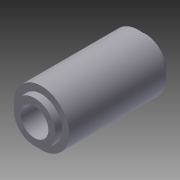
# Autodesk Inventor part: gearbox_standoff
Saved by Autodesk Inventor 2012 (Build 160160000, 160)
## iProperties
Created: 2011-01-16
Part Number: gearbox_standoff
Material: Aluminum-6061
Document SubType Name: Modeling
Designer: Antonella Wilby
Mass: 16.8944 g
Surface Area: 22.1685 cm^2
Volume: 6.23409 cm^3
Density: 2.71 g/cm^3
Author: Antonella Wilby
Autodesk Inventor part; units mm, degrees
ref_plane "YZ Plane" through (0, 0, 0) normal (1, 0, 0) x (0, 1, 0)
ref_plane "XZ Plane" through (0, 0, 0) normal (0, 1, 0) x (-1, 0, 0)
ref_plane "XY Plane" through (0, 0, 0) normal (0, 0, 1) x (1, 0, 0)
sketch "Sketch1" plane through (0, 0, 0) normal (0, 0, 1) x (1, 0, 0)
  circle A0 centre (0, 0) radius 6.35
  circle A1 centre (0, 0) radius 3.175
  dimension "d0" = 12.7
  dimension "d13" = 3.175
  constraints: 2 centre point, 2 coincident
  measures "d0" diameter of A0
  measures "d13" radial gap between concentric circles of A0 A1
extrude "Base" add sketch "Sketch1" along normal mid plane 25.4
sketch "Sketch4" plane through (0, 0, 12.7) normal (0, 0, 1) x (1, 0, 0)
  circle A0 centre (0, 0) radius 6.35 projected
  circle A1 centre (0, 0) radius 4.7625
  dimension "d16" = 9.525
  constraints: 1 centre point, 1 coincident
  measures "d16" diameter of A1
extrude "Extrusion4" cut sketch "Sketch4" against normal blind 1.5875
mirror "Mirror2" about plane through (0, 0, 0) normal (0, 0, 1) of "Extrusion4"
body "Solid2"
